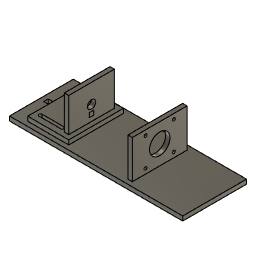
CoilWindingMachine (Autodesk Fusion 360 design; units mm, degrees)
Autodesk Fusion 360 part; units mm, degrees
ref_plane "WorkPlane1" through (0, 0, -21) normal (0, 0, 1) x (1, 0, 0)
ref_plane "WorkPlane2" through (-70, 0, 0) normal (1, 0, 0) x (0, 1, 0)
sketch "nema17_dimensions" plane through (0, 0, 0) normal (1, 0, 0) x (0, 1, 0)
  line L0 (15.5, 15.5) -> (-15.5, 15.5) construction
  line L1 (-15.5, 15.5) -> (-15.5, -15.5) construction
  line L2 (-15.5, -15.5) -> (15.5, -15.5) construction
  line L3 (15.5, -15.5) -> (15.5, 15.5) construction
  line L4 (15.5, 15.5) -> (-15.5, -15.5) construction
  line L5 (-15.5, 15.5) -> (15.5, -15.5) construction
  line L6 (21, 21) -> (-21, 21) construction
  line L7 (-21, 21) -> (-21, -21) construction
  line L8 (-21, -21) -> (21, -21) construction
  line L9 (21, -21) -> (21, 21) construction
  line L10 (21, 21) -> (-21, -21) construction
  line L11 (-21, 21) -> (21, -21) construction
  dimension "d1" = 31
  dimension "d2" = 31
  dimension "d3" = 42
  constraint horizontal L0
  constraint perpendicular L0 L1
  constraint parallel L0 L2
  constraint parallel L1 L3
  constraint coincident L4 origin
  constraint coincident L5 origin
  constraint horizontal L6
  constraint perpendicular L6 L7
  constraint parallel L6 L8
  constraint parallel L7 L9
  constraint coincident L10 origin
  constraint coincident L11 origin
  measures "d1" distance of L1.end L2.end
  measures "d2" distance of L0.end L1.end
  measures "d3" distance of L7.end L8.end
sketch "motor_face" plane through (0, 0, 0) normal (1, 0, 0) x (0, 1, 0)
  circle A0 centre (0, 0) radius 11.25
  circle A1 centre (-15.5, 15.5) radius 1.6
  circle A2 centre (15.5, 15.5) radius 1.6
  circle A3 centre (15.5, -15.5) radius 1.6
  circle A4 centre (-15.5, -15.5) radius 1.6
  line L0 (-30, 21) -> (30, 21)
  line L1 (30, 21) -> (30, -25.8)
  line L2 (30, -25.8) -> (22, -25.8)
  line L3 (22, -25.8) -> (22, -21)
  line L4 (22, -21) -> (5, -21)
  line L5 (5, -21) -> (5, -25.8)
  line L6 (5, -25.8) -> (-5, -25.8)
  line L7 (-5, -25.8) -> (-5, -21)
  line L8 (-5, -21) -> (-22, -21)
  line L9 (-22, -21) -> (-22, -25.8)
  line L10 (-22, -25.8) -> (-30, -25.8)
  line L11 (-30, -25.8) -> (-30, 21)
  point P0 (15.5, 15.5)
  point P1 (-15.5, 15.5)
  point P2 (-15.5, -15.5)
  point P3 (15.5, -15.5)
  dimension "d4" = 22.5
  dimension "d5" = 3.2
  dimension "d6" = 3.2
  dimension "d7" = 3.2
  dimension "d8" = 3.2
  dimension "d9" = 46.8
  dimension "d15" = 60
  constraint coincident A0.centre origin
  constraint coincident P1 A1.centre
  constraint coincident P0 A2.centre
  constraint coincident P3 A3.centre
  constraint coincident P2 A4.centre
  constraint horizontal L0
  constraint perpendicular L0 L1
  constraint perpendicular L1 L2
  constraint perpendicular L0 L3
  constraint perpendicular L3 L4
  constraint perpendicular L2 L5
  constraint perpendicular L5 L6
  constraint perpendicular L2 L7
  constraint perpendicular L7 L8
  constraint perpendicular L6 L9
  constraint perpendicular L7 L10
  constraint perpendicular L10 L11
  measures "d4" diameter of A0
  measures "d5" diameter of A1
  measures "d6" diameter of A2
  measures "d7" diameter of A3
  measures "d8" diameter of A4
  measures "d9" distance of L0.end L1.end
  measures "d15" distance of L0.start L0.end
sketch "base_dimensions" plane through (0, 0, -21) normal (0, 0, 1) x (1, 0, 0)
  line L0 (0, -21) -> (42, -21)
  line L1 (42, -21) -> (42, 21)
  line L2 (42, 21) -> (0, 21)
  line L3 (0, 21) -> (0, -21)
  line L4 (0, -1.5) -> (-12, -1.5)
  line L5 (-12, -1.5) -> (-12, -5)
  line L6 (-12, -5) -> (-32, -5)
  line L7 (-32, -5) -> (-32, 5)
  line L8 (-32, 5) -> (-12, 5)
  line L9 (-12, 5) -> (-12, 1.5)
  line L10 (-12, 1.5) -> (0, 1.5)
  line L11 (-40, -20) -> (-40, 20) construction
  line L12 (-40, -20) -> (-44, -14) construction
  line L13 (-44, -14) -> (-44, 14) construction
  line L14 (-44, 14) -> (-40, 20) construction
  line L15 (-44, -1.5) -> (-49, -1.5) construction
  line L16 (-44, 1.5) -> (-49, 1.5) construction
  line L17 (-49, 1.5) -> (-49, -1.5) construction
  line L18 (-49, -14) -> (-53, -20) construction
  line L19 (-53, -20) -> (-53, 20) construction
  line L20 (-53, 20) -> (-49, 14) construction
  line L21 (-49, 14) -> (-49, -14) construction
  dimension "d16" = 42
  dimension "d17" = 42
  constraint horizontal L0
  constraint vertical L1
  constraint horizontal L2
  constraint vertical L3
  constraint coincident L3 L4.start
  constraint perpendicular L3 L4
  constraint perpendicular L4 L5
  constraint perpendicular L3 L6
  constraint perpendicular L4 L7
  constraint perpendicular L7 L8
  constraint perpendicular L8 L9
  constraint coincident L3 L10.end
  constraint perpendicular L3 L10
  constraint perpendicular L8 L11
  constraint perpendicular L8 L13
  constraint coincident L13 L15.start
  constraint perpendicular L13 L15
  constraint coincident L13 L16.start
  constraint perpendicular L13 L16
  constraint perpendicular L15 L17
  constraint perpendicular L15 L19
  constraint perpendicular L16 L21
  measures "d16" distance of L0.start L0.end
  measures "d17" distance of L0.start L2.end
sketch "base" plane through (0, 0, -21) normal (0, 0, 1) x (1, 0, 0)
  line L0 (0, 30) -> (4.8, 30)
  line L1 (4.8, 30) -> (4.8, 22)
  line L2 (4.8, 22) -> (0, 22)
  line L3 (0, 22) -> (0, 30)
  line L4 (0, 5) -> (4.8, 5)
  line L5 (4.8, 5) -> (4.8, -5)
  line L6 (4.8, -5) -> (0, -5)
  line L7 (0, -5) -> (0, 5)
  line L8 (0, -22) -> (4.8, -22)
  line L9 (4.8, -22) -> (4.8, -30)
  line L10 (4.8, -30) -> (0, -30)
  line L11 (0, -30) -> (0, -22)
  line L12 (65, 35) -> (-125, 35)
  line L13 (-125, 35) -> (-125, -35)
  line L14 (-125, -35) -> (65, -35)
  line L15 (65, -35) -> (65, 35)
  line L16 (-70, 2.5) -> (-120, 2.5)
  line L17 (-120, 2.5) -> (-120, -2.5)
  line L18 (-120, -2.5) -> (-70, -2.5)
  line L19 (-70, -2.5) -> (-70, 2.5)
  circle A0 centre (-95, -22) radius 1.35
  circle A1 centre (-95, 22) radius 1.35
  point P0 (0, 30)
  point P1 (0, 22)
  point P2 (0, 5)
  point P3 (0, -5)
  point P4 (0, -22)
  point P5 (0, -30)
  point P6 (-95, 0)
  point P7 (-95, 22)
  point P8 (-95, -22)
  dimension "d12" = 4.8
  dimension "d13" = 4.8
  dimension "d14" = 4.8
  dimension "d18" = 50
  dimension "d19" = 5
  dimension "d34" = 2.7
  dimension "d35" = 2.7
  constraint horizontal L0
  constraint vertical L1
  constraint horizontal L2
  constraint vertical L3
  constraint coincident P0 L0.start
  constraint horizontal L4
  constraint vertical L5
  constraint horizontal L6
  constraint vertical L7
  constraint coincident P2 L4.start
  constraint horizontal L8
  constraint vertical L9
  constraint horizontal L10
  constraint vertical L11
  constraint coincident P4 L8.start
  constraint horizontal L12
  constraint vertical L13
  constraint horizontal L14
  constraint vertical L15
  constraint horizontal L16
  constraint perpendicular L16 L17
  constraint parallel L16 L18
  constraint parallel L17 L19
  constraint coincident P8 A0.centre
  constraint coincident P7 A1.centre
  measures "d12" distance of P0 L0.end
  measures "d13" distance of P2 L4.end
  measures "d14" distance of P4 L8.end
  measures "d18" distance of L17.end L18.end
  measures "d19" distance of L16.end L17.end
  measures "d34" diameter of A0
  measures "d35" diameter of A1
sketch "slider_base" plane through (0, 0, -21) normal (0, 0, 1) x (1, 0, 0)
  line L0 (-65, -30) -> (-110, -30)
  line L1 (-110, -30) -> (-110, 30)
  line L2 (-110, 30) -> (-65, 30)
  line L3 (-65, 30) -> (-65, -30)
  line L4 (-70, -25) -> (-74.8, -25)
  line L5 (-74.8, -25) -> (-74.8, -17)
  line L6 (-74.8, -17) -> (-70, -17)
  line L7 (-70, -17) -> (-70, -25)
  line L8 (-70, 25) -> (-70, 17)
  line L9 (-70, 17) -> (-74.8, 17)
  line L10 (-74.8, 17) -> (-74.8, 25)
  line L11 (-74.8, 25) -> (-70, 25)
  line L12 (-70, -17) -> (-70, -25)
  line L13 (-70, -25) -> (-74.8, -25)
  line L14 (-74.8, -25) -> (-74.8, -17)
  line L15 (-74.8, -17) -> (-70, -17)
  line L16 (-70, 2.4) -> (-74.8, 2.4)
  line L17 (-74.8, 2.4) -> (-74.8, -2.4)
  line L18 (-74.8, -2.4) -> (-70, -2.4)
  line L19 (-70, -2.4) -> (-70, 2.4)
  line L20 (-79, -2.4) -> (-79, 2.4)
  line L21 (-79, 2.4) -> (-83.8, 2.4)
  line L22 (-83.8, 2.4) -> (-83.8, -2.4)
  line L23 (-83.8, -2.4) -> (-79, -2.4)
  line L24 (-80, -23.75) -> (-104, -23.75)
  line L25 (-80, -20.25) -> (-104, -20.25)
  line L26 (-80, 20.25) -> (-104, 20.25)
  line L27 (-80, 23.75) -> (-104, 23.75)
  arc A0 (-80, -23.75) -> (-80, -20.25) centre (-79.7656, -22) ccw
  arc A1 (-104, -20.25) -> (-104, -23.75) centre (-104, -22) ccw
  arc A2 (-80, 20.25) -> (-80, 23.75) centre (-80, 22) ccw
  arc A3 (-104, 23.75) -> (-104, 20.25) centre (-104, 22) ccw
  point P0 (-72.4, 0)
  point P1 (-95, -22)
  point P2 (-95, 22)
  dimension "d20" = 4.8
  dimension "d21" = 8
  dimension "d22" = 4.8
  dimension "d23" = 8
  dimension "d24" = 4.8
  dimension "d25" = 8
  dimension "d26" = 4.8
  dimension "d27" = 4.8
  dimension "d28" = 4.8
  dimension "d29" = 4.8
  constraint horizontal L0
  constraint vertical L1
  constraint horizontal L2
  constraint vertical L3
  constraint horizontal L4
  constraint vertical L5
  constraint horizontal L6
  constraint vertical L7
  constraint horizontal L9
  constraint vertical L10
  constraint horizontal L11
  constraint vertical L8
  constraint horizontal L13
  constraint vertical L14
  constraint horizontal L15
  constraint vertical L12
  constraint horizontal L16
  constraint perpendicular L16 L17
  constraint parallel L16 L18
  constraint parallel L17 L19
  constraint horizontal L21
  constraint perpendicular L21 L22
  constraint parallel L21 L23
  constraint parallel L20 L22
  constraint parallel L16 L24
  constraint parallel L24 L25
  constraint parallel L25 L26
  constraint parallel L26 L27
  constraint tangent L25 A1
  constraint tangent L27 A2
  constraint tangent L26 A2
  constraint tangent L27 A3
  constraint tangent L26 A3
  measures "d20" distance of L4.start L4.end
  measures "d21" distance of L4.start L6.end
  measures "d22" distance of L9.end L8.end
  measures "d23" distance of L8.start L8.end
  measures "d24" distance of L4.end L4.start
  measures "d25" distance of L6.end L4.start
  measures "d26" distance of L17.end L18.end
  measures "d27" distance of L16.end L17.end
  measures "d28" distance of L20.start L22.end
  measures "d29" distance of L22.end L21.end
sketch "slider_face" plane through (-70, 0, 0) normal (1, 0, 0) x (0, 1, 0)
  line L0 (2.5, -21) -> (2.5, -25)
  line L1 (-2.4, -21) -> (-2.4, -25)
  line L2 (-2.4, -25) -> (2.5, -25)
  line L3 (2.5, -21) -> (2.5, -16.2)
  line L4 (2.5, -16.2) -> (17, -16.2)
  line L5 (17, -16.2) -> (17, -21)
  line L6 (17, -21) -> (25, -21)
  line L7 (25, -21) -> (25, -16.2)
  line L8 (-2.4, -21) -> (-2.4, -16.2)
  line L9 (-2.4, -16.2) -> (-17, -16.2)
  line L10 (-17, -16.2) -> (-17, -21)
  line L11 (-17, -21) -> (-25, -21)
  line L12 (-25, -21) -> (-25, -16.2)
  line L13 (25, -16.2) -> (25, 21)
  line L14 (25, 21) -> (-25, 21)
  line L15 (-25, 21) -> (-25, -16.2)
  circle A0 centre (0, 0) radius 4.5
  line L16 (-2.4, -11.4) -> (2.4, -11.4)
  line L17 (2.4, -11.4) -> (2.4, -6.6)
  line L18 (2.4, -6.6) -> (-2.4, -6.6)
  line L19 (-2.4, -6.6) -> (-2.4, -11.4)
  point P0 (25, -21)
  point P1 (17, -21)
  point P2 (2.5, -21)
  point P3 (-2.4, -21)
  point P4 (-17, -21)
  point P5 (-25, -21)
  point P6 (0, -9)
  dimension "d37" = 4.8
  dimension "d38" = 9
  dimension "d40" = 4.8
  dimension "d41" = 4.8
  constraint coincident P2 L0.start
  constraint vertical L0
  constraint coincident P3 L1.start
  constraint vertical L1
  constraint perpendicular L0 L2
  constraint perpendicular L2 L3
  constraint perpendicular L3 L4
  constraint coincident P1 L5.end
  constraint perpendicular L4 L5
  constraint coincident P0 L6.end
  constraint perpendicular L4 L7
  constraint perpendicular L4 L8
  constraint perpendicular L8 L9
  constraint coincident P4 L10.end
  constraint perpendicular L4 L10
  constraint coincident P5 L11.end
  constraint perpendicular L11 L12
  constraint parallel L7 L13
  constraint perpendicular L12 L14
  constraint perpendicular L14 L15
  constraint coincident A0.centre origin
  constraint horizontal L16
  constraint perpendicular L16 L17
  constraint parallel L16 L18
  constraint parallel L17 L19
  measures "d37" distance of P2 L3.end
  measures "d38" diameter of A0
  measures "d40" distance of L17.end L18.end
  measures "d41" distance of L16.end L17.end
sketch "lock_piece" plane through (0, 0, 0) normal (0, 1, 0) x (1, 0, 0)
  line L0 (-70, 6.6) -> (-83.8, 6.6)
  line L1 (-83.8, 6.6) -> (-83.8, 21)
  line L2 (-83.8, 21) -> (-83.8, 25)
  line L3 (-83.8, 25) -> (-79, 25)
  line L4 (-79, 25) -> (-79, 21)
  line L5 (-79, 21) -> (-79, 16.2)
  line L6 (-70, 16.2) -> (-70, 11.4)
  line L7 (-70, 11.4) -> (-74.8, 11.4)
  line L8 (-74.8, 11.4) -> (-74.8, 16.2)
  line L9 (-79, 16.2) -> (-74.8, 16.2)
  line L10 (-70, 6.6) -> (-70, 11.4)
  point P0 (-70, 6.6)
  point P1 (-70, 11.4)
  point P2 (-70, 16.2)
  point P3 (-79, 21)
  point P4 (-83.8, 21)
  dimension "d42" = 4
  dimension "d43" = 4.8
  constraint coincident P0 L0.start
  constraint horizontal L0
  constraint coincident P4 L1.end
  constraint perpendicular L0 L1
  constraint perpendicular L0 L2
  constraint perpendicular L2 L3
  constraint coincident P3 L4.end
  constraint perpendicular L3 L4
  constraint perpendicular L3 L5
  constraint coincident P2 L6.start
  constraint coincident P1 L6.end
  constraint perpendicular L6 L7
  constraint perpendicular L8 L9
  measures "d42" distance of P4 L2.end
  measures "d43" distance of P1 L7.end
extrude "Extrude1" add sketch "base" against normal blind 4.8 makes body 1
extrude "Extrude2" add sketch "motor_face" along normal blind 4.8 separate body makes body 2
extrude "Extrude3" add sketch "slider_base" along normal blind 4.8 separate body makes body 3
extrude "Extrude4" add sketch "slider_face" against normal blind 4.8 separate body makes body 4
extrude "Extrude5" add sketch "lock_piece" along normal mid plane 4.8 separate body makes body 5
equation "ply_medium = 4.8 mm"
equation "d12 = ply_medium"
equation "d13 = ply_medium"
equation "d14 = ply_medium"
equation "d19 = ply_medium + 0.2 mm"
equation "d20 = ply_medium"
equation "d22 = ply_medium"
equation "d24 = ply_medium"
equation "d26 = ply_medium"
equation "d27 = ply_medium"
equation "d28 = ply_medium"
equation "d29 = ply_medium"
equation "d37 = ply_medium"
equation "d38 = tiny_bearing_od"
equation "tiny_bearing_od = 9 mm"
equation "d40 = ply_medium"
equation "d41 = ply_medium"
equation "d43 = ply_medium"
equation "d44 = -ply_medium"
equation "d46 = ply_medium"
equation "d48 = ply_medium"
equation "d50 = -ply_medium"
equation "d52 = ply_medium / 2"
named bodies: "base", "motor_face", "slider_base", "slider_face", "lock_piece"
